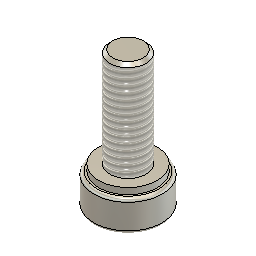
cad_native (Autodesk Fusion 360 archive; units mm, degrees)
design "M3 x 8"
Autodesk Fusion 360 part; units mm, degrees
sketch "Bolt Base" plane through (0, 0, 0) normal (0, 1, 0) x (1, 0, 0)
  circle A0 centre (0, 0) radius 2.75
  line L0 (-0.8424, 1.5134) -> (-1.7318, 0.0271)
  line L1 (-1.7318, 0.0271) -> (-0.8894, -1.4862)
  line L2 (-0.8894, -1.4862) -> (0.8424, -1.5134)
  line L3 (0.8424, -1.5134) -> (1.7318, -0.0271)
  line L4 (1.7318, -0.0271) -> (0.8894, 1.4862)
  line L5 (0.8894, 1.4862) -> (-0.8424, 1.5134)
  dimension "d1" = 5.5
  dimension "d2" = 1.5
  constraint coincident A0.centre origin
  measures "d1" diameter of A0
  measures "d2" distance of A0.centre L5
extrude "Extrude1" add sketch "Bolt Base" along normal blind 3 contours A0 | L0 L1 L2 L3 L4 L5
extrude "Extrude2" cut sketch "Bolt Base" along normal blind 1.5 contours L0 L1 L2 L3 L4 L5
sketch "Bolt thread" plane through (0, 3, 0) normal (0, 1, 0) x (-1, 0, 0)
  circle A0 centre (0, 0) radius 2.75
  circle A1 centre (0, 0) radius 1.5
  circle A2 centre (0, 0) radius 2.35
  dimension "d7" = 3
  dimension "d8" = 4.7
  constraint coincident A0.centre A1.centre
  measures "d7" diameter of A1
  measures "d8" diameter of A2
extrude "Extrude3" cut sketch "Bolt thread" against normal blind 0.5 contours A0
extrude "Extrude4" add sketch "Bolt thread" along normal blind 8 contours A1
fillet "Fillet1" radius 0.25 2 edges at (-2.5639, 2.5, -0.9944) (-2.5639, 0, 0.9944)
thread "Thread1" "ISO Metric profile 3.0 M3x0.5 6g" major diameter 2.927 minor diameter 2.3555 pitch 0.5 angle 60 resizes the face on face at (-1.4925, 5.6667, -0.1494)
chamfer "Chamfer1" distance 0.25 angle 45 1 edges at (1.3645, 11, -0.5292)
chamfer "Chamfer2" distance 0.1 angle 45 6 edges at (1.2871, 0, 0.7703) (-0.0235, 0, 1.4998) (-1.3106, 0, 0.7296) (-1.2871, 0, -0.7703) (0.0235, 0, -1.4998) (1.3106, 0, -0.7296)
equation "d2 = ( 3 / 2 ) * 1 mm"

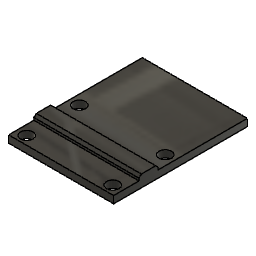
design "Development Board"
Autodesk Fusion 360 part; units mm, degrees
sketch "Sketch1" plane through (0, 0, 0) normal (0, 1, 0) x (1, 0, 0)
  line L0 (0, 0) -> (22, 0)
  line L1 (22, 0) -> (22, 28)
  line L2 (22, 28) -> (0, 28)
  line L3 (0, 28) -> (0, 0)
  line L4 (11, 0) -> (11, 0.5)
  line L5 (11, 0.5) -> (2, 0.5)
  circle A0 centre (2, 1.8) radius 1.3
  line L6 (2, 1.8) -> (2, 12.8)
  circle A1 centre (2, 12.8) radius 1.3
  circle A2 centre (20, 1.8) radius 1.3
  circle A3 centre (20, 12.8) radius 1.3
  line L7 (2, 7.3) -> (22, 7.3)
  line L8 (2, 7.3) -> (0, 7.3)
  line L9 (0, 7.3) -> (0, 5.3)
  line L10 (0, 5.3) -> (22, 5.3)
  line L11 (0, 7.3) -> (0, 9.3)
  line L12 (0, 9.3) -> (22, 9.3)
  dimension "d1" = 22
  dimension "d2" = 28
  dimension "d3" = 0.5
  dimension "d4" = 9
  dimension "d5" = 2.6
  dimension "d6" = 11
  dimension "d7" = 2.6
  dimension "d8" = 2
  dimension "d9" = 2
  constraint horizontal L0
  constraint vertical L1
  constraint horizontal L2
  constraint vertical L3
  constraint coincident L0.start L3.end
  constraint midpoint L0 L4.start
  constraint perpendicular L0 L4
  constraint perpendicular L3 L5
  constraint coincident L5.end A0
  constraint coincident A0.centre L6.start
  constraint perpendicular L5 L6
  constraint coincident L6.end A1.centre
  constraint symmetric L4 A0 A2
  constraint symmetric L4 A1 A3
  constraint midpoint L6 L7.start
  constraint coincident L1 L7.end
  constraint perpendicular L1 L7
  constraint coincident L3 L8.end
  constraint perpendicular L3 L8
  constraint perpendicular L8 L9
  constraint coincident L1 L10.end
  constraint perpendicular L1 L10
  constraint perpendicular L8 L11
  constraint coincident L1 L12.end
  constraint perpendicular L1 L12
  measures "d1" distance of L0.start L0.end
  measures "d2" distance of L0.start L2.end
  measures "d3" distance of L4.start L4.end
  measures "d4" distance of L4.end L5.end
  measures "d5" diameter of A0
  measures "d6" distance of A0.centre L6.end
  measures "d7" diameter of A1
  measures "d8" distance of L8.end L9.end
  measures "d9" distance of L8.end L11.end
extrude "Extrude1" add sketch "Sketch1" against normal blind 1.5 contours L0 L3 L4 L5 A0 L6 L10 | L0 L1 L4 L5 A0 L6 L10 | L3 L6 L8 L9 L10 | L3 L6 L8 L11 L12 | L1 L6 L7 L10 | L1 L2 L3 L12 | L1 L6 L7 L12
extrude "Extrude2" add sketch "Sketch1" along normal blind 1 contours L3 L6 L8 L9 L10 | L3 L6 L8 L11 L12 | L1 L6 L7 L10 | L1 L6 L7 L12
chamfer "Chamfer1" distance 0.5 angle 45 2 edges at (11, 1, -5.3) (11, 1, -9.3)
equation "d4 = ( 18 / 2 ) * 1 mm"
